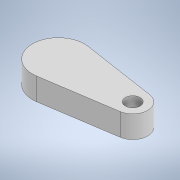
# Autodesk Inventor part: Servo arm
Saved by Autodesk Inventor 2020.4 (Build 244396000, 396)
## iProperties
Created: 2021-05-01
Part Number: Servo arm
Material: Generic
Document SubType Name: Modeling
Designer: armin
Density: 1 g/cm^3
Appearance: Default
Author: armin
Autodesk Inventor part; units mm, degrees
ref_plane "YZ Plane" through (0, 0, 0) normal (1, 0, 0) x (0, 1, 0)
ref_plane "XZ Plane" through (0, 0, 0) normal (0, 1, 0) x (-1, 0, 0)
ref_plane "XY Plane" through (0, 0, 0) normal (0, 0, 1) x (1, 0, 0)
sketch "Sketch1" plane through (0, 0, 0) normal (0, 1, 0) x (-1, 0, 0)
  circle A0 centre (0, 0) radius 3.5
  circle A1 centre (-10, 0) radius 1
  circle A2 centre (-10, 0) radius 2
  line L0 (-10.3, 1.9774) -> (-0.525, 3.4604)
  line L1 (-10.3, -1.9774) -> (-0.525, -3.4604)
  dimension "d0" = 2
  dimension "d1" = 7
  dimension "d2" = 4
  dimension "d3" = 10
  constraints: 4 end point, 4 point on circle, 4 tangent, 3 centre point, 2 coincident
  measures "d0" diameter of A1
  measures "d1" diameter of A0
  measures "d2" diameter of A2
  measures "d3" distance of A1.centre point (0, 0)
extrude "Extrusion1" add sketch "Sketch1" along normal blind 3
body "Solid1"
